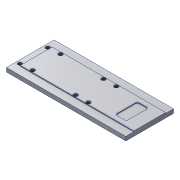
# Autodesk Inventor part: Grundplatte
Saved by Autodesk Inventor 2016 (Build 200138000, 138)
## iProperties
Created: 2015-07-27
Part Number: Grundplatte
Material: Aluminum 6061
Document SubType Name: Modeling
Density: 2.7 g/cm^3
Appearance: Aluminum - Flat
Autodesk Inventor part; units mm, degrees
ref_plane "YZ Plane" through (0, 0, 0) normal (1, 0, 0) x (0, 1, 0)
ref_plane "XZ Plane" through (0, 0, 0) normal (0, 1, 0) x (-1, 0, 0)
ref_plane "XY Plane" through (0, 0, 0) normal (0, 0, 1) x (1, 0, 0)
sketch "Sketch1" plane through (0, 0, 0) normal (0, 0, 1) x (1, 0, 0)
  line L0 (-150, -60) -> (150, -60)
  line L1 (150, -60) -> (150, 60)
  line L2 (150, 60) -> (-150, 60)
  line L3 (-150, 60) -> (-150, -60)
  line L4 (-150, -60) -> (150, 60) construction
  line L5 (150, -60) -> (-150, 60) construction
  point P0 (0, 0)
  dimension "d0" = 300
  dimension "d1" = 120
  constraints: 12 end point, 2 midpoint, 2 parallel, 1 horizontal, 1 perpendicular
  measures "d0" distance of L2.end L1.end
  measures "d1" distance of L1.end L0.end
extrude "Extrusion1" add sketch "Sketch1" along normal blind 12
sketch "Sketch2" plane through (0, 0, 12) normal (0, 0, 1) x (1, 0, 0)
  line L0 (150, -60) -> (-150, -60)
  line L1 (-150, -60) -> (-150, -40)
  line L2 (-150, -40) -> (150, -40)
  line L3 (150, -40) -> (150, -60)
  line L4 (150, 60) -> (-150, 60)
  line L5 (-150, 60) -> (-150, 40)
  line L6 (-150, 40) -> (150, 40)
  line L7 (150, 40) -> (150, 60)
  line L8 (-135, 40) -> (-150, 40)
  line L9 (-150, 40) -> (-150, -40)
  line L10 (-150, -40) -> (-135, -40)
  line L11 (-135, -40) -> (-135, 40)
  line L12 (150, -60) -> (150, 60) projected
  line L13 (-150, -60) -> (150, -60) projected
  line L14 (-150, 60) -> (-150, -60) projected
  line L15 (150, 60) -> (-150, 60) projected
  line L16 (119, 28) -> (91, 28)
  line L17 (91, 28) -> (91, -28)
  line L18 (91, -28) -> (119, -28)
  line L19 (119, -28) -> (119, 28)
  point P0 (0, 0)
  point P1 (91, 0)
  dimension "d4" = 80
  dimension "d5" = 15
  dimension "d6" = 269
  dimension "d7" = 28
  dimension "d8" = 56
  constraints: 32 end point, 8 parallel, 7 collinear, 4 horizontal, 4 perpendicular, 1 horizontal alignment, 1 midpoint, 1 point on line
  measures "d4" distance between parallel lines of L6 L2
  measures "d5" distance between parallel lines of L9 L11
  measures "d6" distance between parallel lines of L14 L19
  measures "d7" distance of L17.end L18.end
  measures "d8" distance of L18.end L16.start
extrude "Extrusion2" cut sketch "Sketch2" against normal blind 2 contours L0 L1 L2 L3 | L9 L6 L11 L2 | L6 L5 L4 L7 | L19 L18 L17 L16
fillet "Fillet1" radius 5 4 edges at (119, 28, 11) (91, 28, 11) (91, -28, 11) (119, -28, 11)
sketch "Sketch3" plane through (0, 0, 12) normal (0, 0, 1) x (1, 0, 0)
  line L0 (-150, -60) -> (-150, 60) projected
  point P0 (0, 0)
  point P1 (-141, -35)
  point P2 (-109, -35)
  point P3 (-109, 35)
  point P4 (-141, 35)
  point P5 (-1, -35)
  point P6 (31, -35)
  point P7 (31, 35)
  point P8 (-1, 35)
  dimension "d12" = 32
  dimension "d13" = 32
  dimension "d14" = 172
  dimension "d15" = 70
  dimension "d16" = 9
  dimension "d17" = 35
  constraints: 6 horizontal alignment, 4 vertical alignment
  measures "d12" distance of point (-109, -35) point (-141, -35)
  measures "d13" distance of point (31, -35) point (-1, -35)
  measures "d14" distance of point (-141, -35) point (31, -35)
  measures "d15" distance of point (-141, 35) point (-141, -35)
  measures "d16" distance from line of L0 point (-141, -35)
  measures "d17" vertical distance of point (0, 0) point (-141, -35)
hole "Hole1" at (-141, -35, 12) at (-109, -35, 12) at (-109, 35, 12) at (-141, 35, 12) at (-1, -35, 12) at (31, -35, 12) at (31, 35, 12) at (-1, 35, 12) direction (0, 0, -1) diameter 5.5 end through all counterbore diameter 10 counterbore depth 7.7 clearance for "Socket Head Cap Screw ISO 4762" size "M5" standard "ISO"
equation "\"d17\" = 0.5 * d15"
body "Solid1"
